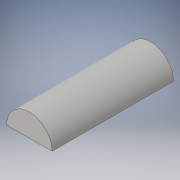
# Autodesk Inventor part: Semi_cilinder
Saved by Autodesk Inventor 2016 (Build 200138000, 138)
## iProperties
Created: 2017-10-18
Part Number: Semi_cilinder
Material: Generic
Document SubType Name: Modeling
Designer: ls769
Density: 1 g/cm^3
Appearance: Default
Author: ls769
Autodesk Inventor part; units mm, degrees
ref_plane "YZ Plane" through (0, 0, 0) normal (1, 0, 0) x (0, 1, 0)
ref_plane "XZ Plane" through (0, 0, 0) normal (0, 1, 0) x (-1, 0, 0)
ref_plane "XY Plane" through (0, 0, 0) normal (0, 0, 1) x (1, 0, 0)
sketch "Sketch2" plane through (0, 0, 0) normal (0, 0, 1) x (1, 0, 0)
  arc A0 (15, 0) -> (-15, 0) centre (0, 0) ccw
  line L0 (-15, 0) -> (-9, 0)
  line L1 (-9, 0) -> (9, 0)
  line L2 (9, 0) -> (15, 0)
  constraints: 6 end point, 3 horizontal, 2 point on circle, 1 centre point, 1 coincident, 1 point on line
extrude "Extrusion2" add sketch "Sketch2" along normal blind 80
body "Solid2"
